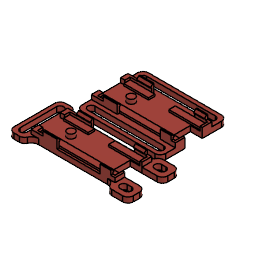
MicrophoneSenzor (Autodesk Fusion 360 design; units mm, degrees)
Autodesk Fusion 360 part; units mm, degrees
note: some values were not read from the file. Set by a fixed rule: which face or edge a step refers to.
sketch "Sketch1" plane through (0, 0, 0) normal (0, 0, 1) x (1, 0, 0)
  line L0 (0, 0) -> (36, 0)
  line L1 (36, 0) -> (36, 15)
  line L2 (36, 15) -> (0, 15)
  line L3 (0, 15) -> (0, 0)
  line L4 (36, 7.5) -> (20, 7.5) construction
  line L5 (36, 12) -> (32, 12)
  line L6 (32, 12) -> (32, 3)
  line L7 (32, 3) -> (36, 3)
  line L8 (36, 3) -> (36, 12)
  line L9 (36, 12) -> (32, 3) construction
  line L10 (32, 12) -> (36, 3) construction
  line L11 (0, 7.5) -> (8, 7.5) construction
  circle A0 centre (8, 7.5) radius 1.8
  point P0 (34, 7.5)
  dimension "d1" = 36
  dimension "d2" = 15
  dimension "d3" = 8
  dimension "d4" = 3.6
  constraint horizontal L0
  constraint vertical L1
  constraint horizontal L2
  constraint vertical L3
  constraint coincident L0.start L3.end
  constraint midpoint L1 L4.start
  constraint perpendicular L1 L4
  constraint horizontal L5
  constraint perpendicular L5 L6
  constraint parallel L5 L7
  constraint parallel L6 L8
  constraint coincident L9 P0
  constraint coincident L10 P0
  constraint coincident L1 L5.start
  constraint coincident L4 P0
  constraint midpoint L3 L11.start
  constraint perpendicular L3 L11
  constraint coincident L11.end A0.centre
  measures "d1" distance of L0.start L0.end
  measures "d2" distance of L0.start L2.end
  measures "d3" distance of L11.start L11.end
  measures "d4" diameter of A0
extrude "Extrude1" add sketch "Sketch1" along normal blind 1.6 contours L0 L1 L2 L3 L5 L6 L7 makes body 1
sketch "Sketch3" plane through (32, 0, 0) normal (1, 0, 0) x (0, 1, 0)
  line L0 (3, 0) -> (12, 0)
  line L1 (12, 0) -> (12, 1.6)
  line L2 (12, 1.6) -> (3, 1.6)
  line L3 (3, 1.6) -> (3, 0)
  circle A0 centre (7.5, 1.6) radius 3
  dimension "d7" = 6
  constraint midpoint L2 A0.centre
  measures "d7" diameter of A0
extrude "Extrude2" add sketch "Sketch3" along normal blind 5.5 contours L0 L2 A0 | L0 A0 | L2 A0 bodies 1
sketch "Sketch4" plane through (0, 0, 1.6) normal (0, 0, 1) x (-1, 0, 0)
  circle A0 centre (-8, -7.5) radius 1.8
  line L0 (-36, -12) -> (-36, -15)
  line L1 (-36, -15) -> (0, -15)
  line L2 (0, -15) -> (0, 0)
  line L3 (0, 0) -> (-36, 0)
  line L4 (-36, 0) -> (-36, -3)
  line L5 (-36, -3) -> (-32, -3)
  line L6 (-32, -3) -> (-32, -4.5)
  line L7 (-32, -4.5) -> (-32, -10.5)
  line L8 (-32, -10.5) -> (-32, -12)
  line L9 (-32, -12) -> (-36, -12)
  line L10 (0, -7.5) -> (-2.5, -7.5) construction
  line L11 (-2.5, -12.5) -> (0, -12.5)
  line L12 (0, -12.5) -> (0, -2.5)
  line L13 (0, -2.5) -> (-2.5, -2.5)
  line L14 (-2.5, -2.5) -> (-2.5, -12.5)
  line L15 (-2.5, -12.5) -> (0, -2.5) construction
  line L16 (0, -12.5) -> (-2.5, -2.5) construction
  circle A1 centre (-2.5, -10) radius 0.05
  circle A2 centre (0, -10) radius 0.05
  circle A3 centre (-2.5, -7.5) radius 0.05
  circle A4 centre (0, -7.5) radius 0.05
  circle A5 centre (-2.5, -5) radius 0.05
  circle A6 centre (0, -5) radius 0.05
  line L17 (-32, -9) -> (-29, -9)
  line L18 (-29, -9) -> (-29, -8.5)
  line L19 (-29, -8.5) -> (-32, -8.5)
  line L20 (-32, -8.5) -> (-32, -9)
  line L21 (-32, -6) -> (-29, -6)
  line L22 (-29, -6) -> (-29, -6.5)
  line L23 (-29, -6.5) -> (-32, -6.5)
  line L24 (-32, -6.5) -> (-32, -6)
  point P0 (-1.25, -7.5)
  dimension "d10" = 0.1
  dimension "d13" = 2.5
  dimension "d14" = 5
  constraint midpoint L2 L10.start
  constraint perpendicular L2 L10
  constraint horizontal L11
  constraint perpendicular L11 L12
  constraint parallel L11 L13
  constraint parallel L12 L14
  constraint coincident L15 P0
  constraint coincident L16 P0
  constraint midpoint L10 P0
  constraint coincident L14 A1.centre
  constraint horizontal L17
  constraint vertical L18
  constraint horizontal L19
  constraint vertical L20
  constraint coincident L7 L17.start
  constraint horizontal L21
  constraint vertical L22
  constraint horizontal L23
  constraint vertical L24
  constraint coincident L7 L21.start
  measures "d10" diameter of A1
extrude "Extrude3" add sketch "Sketch4" along normal blind 0.5 contours L7 L17 L18 L19 L20 | L7 L21 L22 L23 L24 bodies 1
extrude "Extrude4" add sketch "Sketch4" along normal blind 2.5 contours L2 L11 L12 L13 L14 A1 A2 A3 A4 A5 A6 bodies 1
sketch "Sketch5" plane through (0, 0, 1.6) normal (0, 0, 1) x (-1, 0, 0)
  line L0 (-2.5, -2.5) -> (0, -2.5)
  line L1 (0, -2.5) -> (0, 0)
  line L2 (0, 0) -> (-36, 0)
  line L3 (-36, 0) -> (-36, -3)
  line L4 (-36, -3) -> (-32, -3)
  line L5 (-32, -3) -> (-32, -4.5)
  line L6 (-32, -4.5) -> (-32, -6)
  line L7 (-32, -6) -> (-29, -6)
  line L8 (-29, -6) -> (-29, -6.5)
  line L9 (-29, -6.5) -> (-32, -6.5)
  line L10 (-32, -6.5) -> (-32, -8.5)
  line L11 (-32, -8.5) -> (-29, -8.5)
  line L12 (-29, -8.5) -> (-29, -9)
  line L13 (-29, -9) -> (-32, -9)
  line L14 (-32, -9) -> (-32, -10.5)
  line L15 (-32, -10.5) -> (-32, -12)
  line L16 (-32, -12) -> (-36, -12)
  line L17 (-36, -12) -> (-36, -15)
  line L18 (-36, -15) -> (0, -15)
  line L19 (0, -15) -> (0, -12.5)
  line L20 (0, -12.5) -> (-2.5, -12.5)
  line L21 (-2.5, -12.5) -> (-2.5, -10.05)
  arc A0 (-2.5, -10.05) -> (-2.5, -9.95) centre (-2.5, -10) ccw
  line L22 (-2.5, -9.95) -> (-2.5, -7.55)
  arc A1 (-2.5, -7.55) -> (-2.5, -7.45) centre (-2.5, -7.5) ccw
  line L23 (-2.5, -7.45) -> (-2.5, -5.05)
  arc A2 (-2.5, -5.05) -> (-2.5, -4.95) centre (-2.5, -5) ccw
  line L24 (-2.5, -4.95) -> (-2.5, -2.5)
  circle A3 centre (-8, -7.5) radius 1.8
  line L25 (-11.5, -15) -> (-21, -15)
  line L26 (-21, -15) -> (-21, -10.5)
  line L27 (-21, -10.5) -> (-11.5, -10.5)
  line L28 (-11.5, -10.5) -> (-11.5, -15)
  line L29 (-3.5, -14.5) -> (-6, -14.5)
  line L30 (-6, -14.5) -> (-6, -13.5)
  line L31 (-6, -13.5) -> (-3.5, -13.5)
  line L32 (-3.5, -13.5) -> (-3.5, -14.5)
  line L33 (-7.5, -13.5) -> (-7.5, -14.5)
  line L34 (-7.5, -14.5) -> (-10, -14.5)
  line L35 (-10, -14.5) -> (-10, -13.5)
  line L36 (-10, -13.5) -> (-7.5, -13.5)
  line L37 (-10, -1.5) -> (-10, -0.5)
  line L38 (-10, -0.5) -> (-7.5, -0.5)
  line L39 (-7.5, -0.5) -> (-7.5, -1.5)
  line L40 (-7.5, -1.5) -> (-10, -1.5)
  line L41 (-3.5, -0.5) -> (-3.5, -1.5)
  line L42 (-3.5, -1.5) -> (-6, -1.5)
  line L43 (-6, -0.5) -> (-3.5, -0.5)
  line L44 (-6, -1.5) -> (-6, -0.5)
  line L45 (-23, -13) -> (-25.5, -13)
  line L46 (-25.5, -13) -> (-25.5, -12)
  line L47 (-25.5, -12) -> (-23, -12)
  line L48 (-23, -12) -> (-23, -13)
  line L49 (-22, -10.5) -> (-24.5, -10.5)
  line L50 (-24.5, -10.5) -> (-24.5, -9.5)
  line L51 (-24.5, -9.5) -> (-22, -9.5)
  line L52 (-22, -9.5) -> (-22, -10.5)
  line L53 (-22, -3.5) -> (-24.5, -3.5)
  line L54 (-24.5, -3.5) -> (-24.5, -2.5)
  line L55 (-24.5, -2.5) -> (-22, -2.5)
  line L56 (-22, -2.5) -> (-22, -3.5)
  line L57 (-24.5, -1) -> (-22, -1)
  line L58 (-22, -1) -> (-22, -2)
  line L59 (-22, -2) -> (-24.5, -2)
  line L60 (-24.5, -2) -> (-24.5, -1)
  line L61 (-14, -6.5) -> (-18, -6.5)
  line L62 (-18, -6.5) -> (-18, -1.5)
  line L63 (-18, -1.5) -> (-14, -1.5)
  line L64 (-14, -1.5) -> (-14, -6.5)
  dimension "d19" = 9.5
  dimension "d20" = 4.5
  dimension "d21" = 2.5
  dimension "d22" = 1
  dimension "d23" = 2.5
  dimension "d24" = 1
  dimension "d25" = 2.5
  dimension "d26" = 1
  dimension "d27" = 2.5
  dimension "d28" = 1
  dimension "d29" = 2.5
  dimension "d30" = 1
  dimension "d31" = 2.5
  dimension "d32" = 1
  dimension "d33" = 2.5
  dimension "d34" = 1
  dimension "d35" = 2.5
  dimension "d36" = 1
  dimension "d37" = 4
  dimension "d38" = 5
  constraint horizontal L25
  constraint vertical L26
  constraint horizontal L27
  constraint vertical L28
  constraint horizontal L29
  constraint vertical L30
  constraint horizontal L31
  constraint vertical L32
  constraint horizontal L34
  constraint vertical L35
  constraint horizontal L36
  constraint vertical L33
  constraint horizontal L42
  constraint vertical L44
  constraint horizontal L43
  constraint vertical L41
  constraint horizontal L40
  constraint vertical L37
  constraint horizontal L38
  constraint vertical L39
  constraint horizontal L45
  constraint vertical L46
  constraint horizontal L47
  constraint vertical L48
  constraint horizontal L49
  constraint vertical L50
  constraint horizontal L51
  constraint vertical L52
  constraint horizontal L53
  constraint vertical L54
  constraint horizontal L55
  constraint vertical L56
  constraint horizontal L59
  constraint vertical L60
  constraint horizontal L57
  constraint vertical L58
  constraint horizontal L61
  constraint vertical L62
  constraint horizontal L63
  constraint vertical L64
  measures "d19" distance of L25.start L25.end
  measures "d20" distance of L25.start L27.end
  measures "d21" distance of L29.start L29.end
  measures "d22" distance of L29.start L31.end
  measures "d23" distance of L33.end L34.end
  measures "d24" distance of L33.end L33.start
  measures "d25" distance of L41.end L42.end
  measures "d26" distance of L41.end L41.start
  measures "d27" distance of L37.start L39.end
  measures "d28" distance of L39.end L38.end
  measures "d29" distance of L45.end L45.start
  measures "d30" distance of L45.start L47.end
  measures "d31" distance of L49.end L49.start
  measures "d32" distance of L49.start L51.end
  measures "d33" distance of L53.end L53.start
  measures "d34" distance of L53.start L55.end
  measures "d35" distance of L59.end L58.end
  measures "d36" distance of L58.end L57.end
  measures "d37" distance of L61.start L61.end
  measures "d38" distance of L61.start L63.end
extrude "Extrude5" add sketch "Sketch5" along normal blind 10.5 contours L18 L25 L26 L27 L28 bodies 1
extrude "Extrude6" add sketch "Sketch5" along normal blind 0.5 contours L29 L30 L31 L32 | L33 L34 L35 L36 | L37 L38 L39 L40 | L41 L42 L43 L44 | L45 L46 L47 L48 | L49 L50 L51 L52 | L53 L54 L55 L56 | L57 L58 L59 L60 bodies 1
extrude "Extrude7" add sketch "Sketch5" along normal blind 1 contours L61 L62 L63 L64 bodies 1
sketch "Sketch6" plane through (0, 0, 4.1) normal (0, 0, 1) x (-1, 0, 0)
  line L0 (0, -9.95) -> (0, -7.55)
  arc A0 (0, -7.45) -> (0, -7.55) centre (0, -7.5) ccw
  line L1 (0, -7.45) -> (0, -5.05)
  arc A1 (0, -4.95) -> (0, -5.05) centre (0, -5) ccw
  line L2 (0, -4.95) -> (0, -2.5)
  line L3 (0, -2.5) -> (-2.5, -2.5)
  line L4 (-2.5, -2.5) -> (-2.5, -4.95)
  arc A2 (-2.5, -5.05) -> (-2.5, -4.95) centre (-2.5, -5) ccw
  line L5 (-2.5, -5.05) -> (-2.5, -7.45)
  arc A3 (-2.5, -7.55) -> (-2.5, -7.45) centre (-2.5, -7.5) ccw
  line L6 (-2.5, -7.55) -> (-2.5, -9.95)
  arc A4 (-2.5, -10.05) -> (-2.5, -9.95) centre (-2.5, -10) ccw
  line L7 (-2.5, -10.05) -> (-2.5, -12.5)
  line L8 (-2.5, -12.5) -> (0, -12.5)
  line L9 (0, -12.5) -> (0, -10.05)
  arc A5 (0, -9.95) -> (0, -10.05) centre (0, -10) ccw
  line L10 (-1, -11.5) -> (-1.5, -11.5)
  line L11 (-1.5, -11.5) -> (-1.5, -11)
  line L12 (-1.5, -11) -> (-1, -11)
  line L13 (-1, -11) -> (-1, -11.5)
  line L14 (-1, -9) -> (-1.5, -9)
  line L15 (-1.5, -9) -> (-1.5, -8.5)
  line L16 (-1.5, -8.5) -> (-1, -8.5)
  line L17 (-1, -8.5) -> (-1, -9)
  line L18 (-1, -6.5) -> (-1.5, -6.5)
  line L19 (-1.5, -6.5) -> (-1.5, -6)
  line L20 (-1.5, -6) -> (-1, -6)
  line L21 (-1, -6) -> (-1, -6.5)
  line L22 (-1, -4) -> (-1.5, -4)
  line L23 (-1.5, -4) -> (-1.5, -3.5)
  line L24 (-1.5, -3.5) -> (-1, -3.5)
  line L25 (-1, -3.5) -> (-1, -4)
  dimension "d47" = 0
  dimension "d48" = 7.5
  constraint horizontal L10
  constraint vertical L11
  constraint horizontal L12
  constraint vertical L13
extrude "Extrude8" add sketch "Sketch6" along normal blind 1.5 contours L10 L11 L12 L13 | L14 L15 L16 L17 | L18 L19 L20 L21 | L22 L23 L24 L25 bodies 1
sketch "Sketch7" plane through (1, 0, 0) normal (-1, 0, 0) x (0, -1, 0)
  line L0 (-11.5, 4.1) -> (-11, 4.1)
  line L1 (-11, 4.1) -> (-11, 5.6)
  line L2 (-11, 5.6) -> (-11.5, 5.6)
  line L3 (-11.5, 5.6) -> (-11.5, 4.1)
  line L4 (-11, 5.6) -> (-11.5, 5.6)
  line L5 (-11.5, 5.6) -> (-11.5, 5.1)
  line L6 (-11.5, 5.1) -> (-11, 5.1)
  line L7 (-11, 5.1) -> (-11, 5.6)
  line L8 (-9, 5.6) -> (-9, 5.1)
  line L9 (-9, 5.1) -> (-8.5, 5.1)
  line L10 (-8.5, 5.6) -> (-9, 5.6)
  line L11 (-8.5, 5.1) -> (-8.5, 5.6)
  line L12 (-6.5, 5.6) -> (-6.5, 5.1)
  line L13 (-6.5, 5.1) -> (-6, 5.1)
  line L14 (-6, 5.6) -> (-6.5, 5.6)
  line L15 (-6, 5.1) -> (-6, 5.6)
  line L16 (-4, 5.6) -> (-4, 5.1)
  line L17 (-4, 5.1) -> (-3.5, 5.1)
  line L18 (-3.5, 5.6) -> (-4, 5.6)
  line L19 (-3.5, 5.1) -> (-3.5, 5.6)
  dimension "d51" = 0.5
  dimension "d54" = 7.5
  dimension "d55" = 0
  constraint horizontal L4
  constraint vertical L5
  constraint horizontal L6
  constraint vertical L7
  constraint coincident L1.end L2.start
  measures "d51" distance of L1.end L6.end
extrude "Extrude9" add sketch "Sketch7" along normal blind 7 contours L1 L2 L3 L4 L5 L6 L7 | L8 L9 L10 L11 | L12 L13 L14 L15 | L16 L17 L18 L19 bodies 1
sketch "Sketch8" plane through (0, 0, 12.1) normal (0, 0, 1) x (-1, 0, 0)
  line L0 (-11.5, -10.5) -> (-21, -10.5)
  line L1 (-21, -10.5) -> (-21, -15)
  line L2 (-21, -15) -> (-11.5, -15)
  line L3 (-11.5, -15) -> (-11.5, -10.5)
  circle A0 centre (-12.5, -14) radius 1
  constraint tangent L2 A0
extrude "Extrude10" add sketch "Sketch8" along normal blind 1 contours A0 bodies 1
sketch "Sketch10" plane through (0, 0, 0) normal (0, 0, 1) x (1, 0, 0)
  line L0 (-2, 17) -> (37, 17)
  line L1 (37, 17) -> (37, -2)
  line L2 (37, -2) -> (-2, -2)
  line L3 (-2, -2) -> (-2, 17)
  line L4 (37, 11.5) -> (31.5, 11.5)
  line L5 (31.5, 11.5) -> (31.5, 3.5)
  line L6 (31.5, 3.5) -> (37, 3.5)
  line L7 (37, 3.5) -> (37, 11.5)
  constraint horizontal L0
  constraint vertical L1
  constraint horizontal L2
  constraint vertical L3
  constraint horizontal L4
  constraint vertical L5
  constraint horizontal L6
  constraint vertical L7
  constraint coincident L1 L4.start
sketch "Sketch11" plane through (0, 0, 0) normal (0, 0, -1) x (1, 0, 0)
  circle A0 centre (8, -7.5) radius 1.8
  line L0 (36, -15) -> (36, -12)
  line L1 (36, -12) -> (32, -12)
  line L2 (32, -12) -> (32, -10.0377)
  line L3 (32, -10.0377) -> (32, -4.9623)
  line L4 (32, -4.9623) -> (32, -3)
  line L5 (32, -3) -> (36, -3)
  line L6 (36, -3) -> (36, 0)
  line L7 (36, 0) -> (0, 0)
  line L8 (0, 0) -> (0, -15)
  line L9 (0, -15) -> (36, -15)
  circle A1 centre (1.25, -3.75) radius 0.3536
  circle A2 centre (1.25, -6.25) radius 0.3536
  circle A3 centre (1.25, -8.75) radius 0.3536
  circle A4 centre (1.25, -11.25) radius 0.3536
  circle A5 centre (14.75, -13.75) radius 0.3536
  circle A6 centre (16.25, -13.75) radius 0.3536
  circle A7 centre (17.75, -13.75) radius 0.3536
  circle A8 centre (29.25, -6.25) radius 0.3536
  circle A9 centre (29.25, -8.75) radius 0.3536
extrude "Extrude11" add sketch "Sketch11" along normal blind 0.5 draft -30 contours A1 | A2 | A3 | A4 | A5 | A6 | A7 | A8 | A9 bodies 1
move_body "Move1" bodies 1 to x (1, 0, 0) y (0, 1, 0) z (0, 0, 1) at (0, 0, 1)
extrude "Extrude12" add sketch "Sketch10" against normal blind 2.5 separate body contours L0 L1 L2 L3 L4 L5 L6 makes body 2
sketch "Sketch12" plane through (0, 0, 0) normal (0, 0, 1) x (-1, 0, 0)
  line L0 (-31.5, -3.5) -> (-31.5, -11.5)
  line L1 (-31.5, -11.5) -> (-37, -11.5)
  line L2 (-37, -11.5) -> (-37, -17)
  line L3 (-37, -17) -> (2, -17)
  line L4 (2, -17) -> (2, 2)
  line L5 (2, 2) -> (-37, 2)
  line L6 (-37, 2) -> (-37, -3.5)
  line L7 (-37, -3.5) -> (-31.5, -3.5)
  line L8 (-36, -15) -> (-21, -15)
  line L9 (-21, -15) -> (-21, -12)
  line L10 (-21, -12) -> (-36, -12)
  line L11 (-36, -12) -> (-36, -15)
  line L12 (-36, 0) -> (-21, 0)
  line L13 (-21, -3) -> (-36, -3)
  line L14 (-36, -3) -> (-36, 0)
  line L15 (0, 0) -> (-21, 0)
  line L16 (-21, -3) -> (0, -3)
  line L17 (0, -3) -> (0, 0)
  line L18 (0, -15) -> (-11.5, -15)
  line L19 (-11.5, -15) -> (-11.5, -12)
  line L20 (-11.5, -12) -> (0, -12)
  line L21 (0, -12) -> (0, -15)
  circle A0 centre (-8, -7.5) radius 1.75
  dimension "d64" = 3.5
  constraint horizontal L8
  constraint vertical L9
  constraint horizontal L10
  constraint vertical L11
  constraint horizontal L12
  constraint horizontal L13
  constraint vertical L14
  constraint horizontal L15
  constraint horizontal L16
  constraint vertical L17
  constraint coincident L15.start L17.end
  constraint horizontal L18
  constraint vertical L19
  constraint horizontal L20
  constraint vertical L21
  measures "d64" diameter of A0
extrude "Extrude13" add sketch "Sketch12" along normal blind 1 contours L8 L9 L10 L11 | L12 L13 L14 L15 L16 L17 | L18 L19 L20 L21 bodies 2
sketch "Sketch13" plane through (0, 0, 0) normal (0, 0, 1) x (-1, 0, 0)
  line L0 (-36, -12) -> (-21, -12)
  line L1 (-21, -12) -> (-21, -15)
  line L2 (-21, -15) -> (-36, -15)
  line L3 (-36, -15) -> (-36, -12)
  line L4 (0, -12) -> (0, -15)
  line L5 (0, -15) -> (-11.5, -15)
  line L6 (-11.5, -15) -> (-11.5, -12)
  line L7 (-11.5, -12) -> (0, -12)
  line L8 (-36, -3) -> (-36, 0)
  line L9 (-36, 0) -> (0, 0)
  line L10 (0, 0) -> (0, -3)
  line L11 (0, -3) -> (-36, -3)
  line L12 (-31.5, -3.5) -> (-31.5, -11.5)
  line L13 (-31.5, -11.5) -> (-37, -11.5)
  line L14 (-37, -11.5) -> (-37, -17)
  line L15 (-37, -17) -> (2, -17)
  line L16 (2, -17) -> (2, 2)
  line L17 (2, 2) -> (-37, 2)
  line L18 (-37, 2) -> (-37, -3.5)
  line L19 (-37, -3.5) -> (-31.5, -3.5)
  line L20 (-35, 2) -> (-30, 2)
  line L21 (-30, 2) -> (-30, 0)
  line L22 (-30, 0) -> (-35, 0)
  line L23 (-35, 0) -> (-35, 2)
  line L24 (-10, 2) -> (-3.5, 2)
  line L25 (-3.5, 2) -> (-3.5, 0)
  line L26 (-3.5, 0) -> (-10, 0)
  line L27 (-10, 0) -> (-10, 2)
  line L28 (2, -7.5) -> (-32, -7.5) construction
  line L29 (-3.5, -17) -> (-3.5, -15)
  line L30 (-3.5, -15) -> (-10, -15)
  line L31 (-10, -17) -> (-3.5, -17)
  line L32 (-10, -15) -> (-10, -17)
  line L33 (-35, -15) -> (-35, -17)
  line L34 (-35, -17) -> (-30, -17)
  line L35 (-30, -15) -> (-35, -15)
  line L36 (-30, -17) -> (-30, -15)
  constraint horizontal L20
  constraint vertical L21
  constraint horizontal L22
  constraint vertical L23
  constraint coincident L9 L21.end
  constraint coincident L17 L20.start
  constraint horizontal L24
  constraint vertical L25
  constraint horizontal L26
  constraint vertical L27
  constraint coincident L9 L25.end
  constraint coincident L17 L24.start
  constraint midpoint L16 L28.start
  constraint perpendicular L12 L28
  constraint symmetric L20.start L28 L33.end
  constraint symmetric L20.end L28 L34.end
  constraint symmetric L21.end L28 L35.start
  constraint symmetric L22.end L28 L33.start
  constraint symmetric L24.start L28 L31.start
  constraint symmetric L24.end L28 L29.start
  constraint symmetric L25.end L28 L29.end
  constraint symmetric L26.end L28 L30.end
extrude "Extrude14" add sketch "Sketch13" sketch "Sketch12" along normal blind 4 contours L2 L15 L33 L34 L35 L36 | L5 L15 L29 L30 L31 L32 | L9 L17 L24 L25 L26 L27 | L9 L17 L20 L21 L22 L23 of sketch 2 contours A0 bodies 2
sketch "Sketch14" plane through (0, 0, 4) normal (0, 0, 1) x (-1, 0, 0)
  line L0 (-10, 0) -> (-3.5, 0)
  line L1 (-3.5, 0) -> (-3.5, 2)
  line L2 (-3.5, 2) -> (-10, 2)
  line L3 (-10, 2) -> (-10, 0)
  line L4 (-3.5, -0.5) -> (-10, -0.5)
  line L5 (-10, -0.5) -> (-10, 0)
  line L6 (-10, 0) -> (-3.5, 0)
  line L7 (-3.5, 0) -> (-3.5, -0.5)
  line L8 (-35, 0) -> (-30, 0)
  line L9 (-30, 0) -> (-30, -0.5)
  line L10 (-30, -0.5) -> (-35, -0.5)
  line L11 (-35, -0.5) -> (-35, 0)
  line L12 (-32, 0) -> (-32, -15) construction
  line L13 (-32, -15) -> (-32, -7.5) construction
  line L14 (-5, -7.5) -> (-32, -7.5) construction
  line L15 (-10, -15) -> (-3.5, -15)
  line L16 (-3.5, -15) -> (-3.5, -14.5)
  line L17 (-3.5, -14.5) -> (-10, -14.5)
  line L18 (-10, -14.5) -> (-10, -15)
  line L19 (-35, -15) -> (-30, -15)
  line L20 (-30, -15) -> (-30, -14.5)
  line L21 (-35, -14.5) -> (-35, -15)
  line L22 (-30, -14.5) -> (-35, -14.5)
  constraint horizontal L4
  constraint vertical L5
  constraint horizontal L6
  constraint vertical L7
  constraint coincident L0.start L3.end
  constraint horizontal L8
  constraint vertical L9
  constraint horizontal L10
  constraint vertical L11
  constraint coincident L8 L12.start
  constraint perpendicular L10 L12
  constraint midpoint L12 L13.end
  constraint perpendicular L13 L14
  constraint symmetric L4.start L14 L16.end
  constraint symmetric L4.end L14 L17.end
  constraint symmetric L0.start L14 L15.start
  constraint symmetric L0.end L14 L15.end
  constraint symmetric L8.start L14 L19.start
  constraint symmetric L8.end L14 L19.end
  constraint symmetric L9.end L14 L20.end
  constraint symmetric L10.end L14 L21.start
extrude "Extrude15" add sketch "Sketch14" against normal blind 1.3 contours L0 L4 L5 L6 L7 | L8 L9 L10 L11 | L15 L16 L17 L18 | L19 L20 L21 L22 bodies 2
chamfer "Chamfer1" distance 1 angle 45 4 edges at (6.75, 14.5, 4) (6.75, 0.5, 4) (32.5, 0.5, 4) (32.5, 14.5, 4) on bodies 2
sketch "Sketch15" plane through (0, 0, 0) normal (0, 0, 1) x (-1, 0, 0)
  line L0 (0, -2.5) -> (2, -2.5)
  line L1 (2, -2.5) -> (2, 2)
  line L2 (2, 2) -> (0, 2)
  line L3 (0, 0) -> (0, -2.5)
  line L4 (-3.5, 2) -> (0, 2)
  line L5 (0, 0) -> (-3.5, 0)
  line L6 (-3.5, 0) -> (-3.5, 2)
  line L7 (0, -12.5) -> (2, -12.5)
  line L8 (2, -12.5) -> (2, -17)
  line L9 (2, -17) -> (0, -17)
  line L10 (0, -15) -> (0, -12.5)
  line L11 (-3.5, -17) -> (0, -17)
  line L12 (0, -15) -> (-3.5, -15)
  line L13 (-3.5, -15) -> (-3.5, -17)
  line L14 (-35, 2) -> (-37, 2)
  line L15 (-37, 2) -> (-37, 0)
  line L16 (-36, 0) -> (-35, 0)
  line L17 (-35, 0) -> (-35, 2)
  line L18 (-37, -3.5) -> (-36, -3.5)
  line L19 (-36, -3.5) -> (-36, 0)
  line L20 (-37, 0) -> (-37, -3.5)
  line L21 (-37, -11.5) -> (-36, -11.5)
  line L22 (-36, -11.5) -> (-36, -15)
  line L23 (-37, -15) -> (-37, -11.5)
  line L24 (-35, -17) -> (-37, -17)
  line L25 (-37, -17) -> (-37, -15)
  line L26 (-36, -15) -> (-35, -15)
  line L27 (-35, -15) -> (-35, -17)
  constraint horizontal L0
  constraint vertical L1
  constraint horizontal L2
  constraint vertical L3
  constraint horizontal L4
  constraint horizontal L5
  constraint vertical L6
  constraint coincident L3.start L5.start
  constraint coincident L5 L3.start
  constraint horizontal L7
  constraint vertical L8
  constraint horizontal L9
  constraint vertical L10
  constraint horizontal L11
  constraint horizontal L12
  constraint vertical L13
  constraint horizontal L14
  constraint vertical L15
  constraint horizontal L16
  constraint vertical L17
  constraint horizontal L18
  constraint vertical L19
  constraint vertical L20
  constraint horizontal L21
  constraint vertical L22
  constraint vertical L23
  constraint horizontal L24
  constraint vertical L25
  constraint horizontal L26
  constraint vertical L27
extrude "Extrude16" add sketch "Sketch15" along normal blind 2 bodies 2
copy_body "CopyPasteBodies1" bodies 2 makes body 3
sketch "Sketch16" plane through (0, 0, -2.5) normal (0, 0, -1) x (1, 0, 0)
  line L0 (31.5, -11.5) -> (31.5, -3.5)
  line L1 (31.5, -3.5) -> (37, -3.5)
  line L2 (37, -3.5) -> (37, 2)
  line L3 (37, 2) -> (-2, 2)
  line L4 (-2, 2) -> (-2, -17)
  line L5 (-2, -17) -> (37, -17)
  line L6 (37, -17) -> (37, -11.5)
  line L7 (37, -11.5) -> (31.5, -11.5)
  line L8 (-2, 2) -> (37, 2) construction
  line L9 (37, -3.5) -> (37, -17) construction
  line L10 (37, -17) -> (-2, -17) construction
  line L11 (-2, -17) -> (-2, 2) construction
  line L12 (17.5, -7.5) -> (-5.5, -7.5) construction
  line L13 (-5.5, -7.5) -> (42.5, -7.5) construction
  line L14 (42.5, -7.5) -> (42.5, -15.5) construction
  line L15 (42.5, -15.5) -> (42.5, 0.5) construction
  line L16 (-9, -7.5) -> (-9, -17)
  line L17 (-2, -17) -> (-2, -7.5)
  line L18 (-9, -7.5) -> (-9, 2)
  line L19 (-6.5, 4.5) -> (-2, 4.5)
  line L20 (-2, 2) -> (-2, -7.5)
  line L21 (-7.15, 1) -> (-7.15, -16)
  arc A0 (-7.15, -16) -> (-3.85, -16) centre (-5.5, -16) ccw
  line L22 (-3.85, -16) -> (-3.85, 1)
  arc A1 (-3.85, 1) -> (-7.15, 1) centre (-5.5, 1) ccw
  line L23 (-5.5, 1) -> (-5.5, -16) construction
  line L24 (44, -3.5) -> (38.5, -3.5)
  line L25 (38.5, 4.5) -> (44, 4.5)
  line L26 (46.5, 2) -> (46.5, -1)
  line L27 (46.5, -3.5) -> (38.5, 4.5) construction
  line L28 (38.5, -3.5) -> (46.5, 4.5) construction
  line L29 (46.5, -14) -> (46.5, -17)
  line L30 (46.5, -19.5) -> (38.5, -11.5) construction
  line L31 (38.5, -19.5) -> (46.5, -11.5) construction
  line L32 (38.5, 4.5) -> (-2, 4.5)
  line L33 (37, -3.5) -> (38.5, -3.5)
  arc A2 (-9, -17) -> (-6.5, -19.5) centre (-6.5, -17) ccw
  arc A3 (-6.5, 4.5) -> (-9, 2) centre (-6.5, 2) ccw
  arc A4 (46.5, 2) -> (44, 4.5) centre (44, 2) ccw
  arc A5 (44, -3.5) -> (46.5, -1) centre (44, -1) ccw
  arc A6 (46.5, -14) -> (44, -11.5) centre (44, -14) ccw
  arc A7 (44, -19.5) -> (46.5, -17) centre (44, -17) ccw
  line L34 (44, -11.5) -> (37, -11.5)
  line L35 (44, -19.5) -> (-6.5, -19.5)
  line L36 (42.5, 2.15) -> (40.5, 2.15)
  arc A8 (40.5, 2.15) -> (40.5, -1.15) centre (40.5, 0.5) ccw
  line L37 (40.5, -1.15) -> (42.5, -1.15)
  arc A9 (42.5, -1.15) -> (42.5, 2.15) centre (42.5, 0.5) ccw
  line L38 (42.5, 0.5) -> (40.5, 0.5) construction
  line L39 (42.5, -13.85) -> (40.5, -13.85)
  arc A10 (40.5, -13.85) -> (40.5, -17.15) centre (40.5, -15.5) ccw
  line L40 (40.5, -17.15) -> (42.5, -17.15)
  arc A11 (42.5, -17.15) -> (42.5, -13.85) centre (42.5, -15.5) ccw
  arc A12 (42.5, -17.15) -> (42.5, -13.85) centre (42.5, -15.5) ccw
  arc A13 (42.5, -1.15) -> (42.5, 2.15) centre (42.5, 0.5) ccw
  point P0 (-5.5, -7.5)
  point P1 (42.5, 0.5)
  point P2 (42.5, -15.5)
  dimension "d74" = 3.3
  dimension "d75" = 17
  dimension "d76" = 7
  dimension "d77" = 7
  dimension "d78" = 3.3
  dimension "d79" = 3.3
  dimension "d80" = 8
  dimension "d81" = 8
  dimension "d84" = 2.5
  constraint horizontal L8
  constraint vertical L9
  constraint horizontal L10
  constraint vertical L11
  constraint coincident L5.end L6.start
  constraint coincident L3.end L4.start
  constraint perpendicular L4 L12
  constraint perpendicular L9 L13
  constraint perpendicular L13 L14
  constraint perpendicular L13 L15
  constraint vertical L16
  constraint vertical L17
  constraint midpoint L4 L17.end
  constraint vertical L18
  constraint horizontal L19
  constraint vertical L20
  constraint tangent L21 A0
  constraint tangent A0 L22
  constraint parallel L21 L22
  constraint tangent L22 A1
  constraint tangent L21 A1
  constraint perpendicular L12 L23
  constraint coincident P0 L12.end
  constraint midpoint L23 P0
  constraint coincident P2 L14.end
  constraint coincident P1 L15.end
  constraint horizontal L24
  constraint parallel L24 L25
  constraint coincident L27 P1
  constraint coincident L28 P1
  constraint coincident L30 P2
  constraint coincident L31 P2
  constraint perpendicular L20 L32
  constraint coincident L1.end L2.start
  constraint tangent L16 A2
  constraint tangent L18 A3
  constraint tangent L19 A3
  constraint equal A2 A3
  constraint coincident L28.end L26
  constraint coincident L28.end L25
  constraint tangent L26 A4
  constraint tangent L25 A4
  constraint equal A2 A4
  constraint coincident L27.start L24
  constraint coincident L27.start L26
  constraint tangent L24 A5
  constraint tangent L26 A5
  constraint equal A2 A5
  constraint coincident L31.end L29
  constraint tangent L29 A6
  constraint equal A2 A6
  constraint coincident L30.start L29
  constraint tangent L29 A7
  constraint equal A2 A7
  constraint coincident L6.end L7.start
  constraint tangent A2 L35
  constraint tangent L36 A8
  constraint tangent A8 L37
  constraint parallel L36 L37
  constraint tangent L37 A9
  constraint tangent L36 A9
  constraint horizontal L38
  constraint tangent L39 A10
  constraint tangent A10 L40
  constraint parallel L39 L40
  constraint tangent L40 A11
  constraint tangent L39 A11
  measures "d74" diameter of A0
  measures "d75" distance of A1.centre A0.centre
  measures "d76" distance of L16 L17
  measures "d77" distance of L18 L20
  measures "d78" diameter of A12
  measures "d79" diameter of A13
  measures "d80" distance of L30.end L31.end
  measures "d81" distance of L31.start L30.end
  measures "d84" radius of A2
extrude "Extrude17" add sketch "Sketch16" against normal blind 2.5 contours L2 L3 L4 L5 L6 L16 L17 L18 L19 L20 L24 L25 L26 L29 L32 L33 A2 A3 A4 A5 A6 A7 L34 L35 bodies 2
sketch "Sketch17" plane through (0, 0, -2.5) normal (0, 0, -1) x (1, 0, 0)
  line L0 (31.5, -11.5) -> (31.5, -3.5)
  line L1 (31.5, -3.5) -> (37, -3.5)
  line L2 (37, -3.5) -> (37, 2)
  line L3 (37, 2) -> (-2, 2)
  line L4 (-2, 2) -> (-2, -17)
  line L5 (-2, -17) -> (37, -17)
  line L6 (37, -17) -> (37, -11.5)
  line L7 (37, -11.5) -> (31.5, -11.5)
  line L8 (-2, -17) -> (37, -17) construction
  line L9 (37, -17) -> (37, 2) construction
  line L10 (37, 2) -> (-2, 2) construction
  line L11 (-2, 2) -> (-2, -17) construction
  line L12 (37, -7.5) -> (-2, -7.5) construction
  line L13 (17.5, -7.5) -> (17.5, -17) construction
  line L14 (17.5, 2) -> (17.5, -7.5) construction
  line L15 (17.5, -7.5) -> (17.5, -19.5) construction
  line L16 (17.5, -19.5) -> (17.5, 4.5) construction
  line L17 (-2, 2) -> (37, 2)
  line L18 (37, 2) -> (37, 5.5)
  line L19 (34.5, 8) -> (0.5, 8)
  line L20 (-2, 5.5) -> (-2, 2)
  line L21 (-2, -17) -> (37, -17)
  line L22 (37, -17) -> (37, -20.5)
  line L23 (34.5, -23) -> (0.5, -23)
  line L24 (-2, -20.5) -> (-2, -17)
  line L25 (1.5, -21.15) -> (33.5, -21.15)
  arc A0 (33.5, -21.15) -> (33.5, -17.85) centre (33.5, -19.5) ccw
  line L26 (33.5, -17.85) -> (1.5, -17.85)
  arc A1 (1.5, -17.85) -> (1.5, -21.15) centre (1.5, -19.5) ccw
  line L27 (1.5, -19.5) -> (33.5, -19.5) construction
  line L28 (1.5, 6.15) -> (33.5, 6.15)
  arc A2 (33.5, 2.85) -> (33.5, 6.15) centre (33.5, 4.5) ccw
  arc A3 (1.5, 6.15) -> (1.5, 2.85) centre (1.5, 4.5) ccw
  line L29 (33.5, 2.85) -> (1.5, 2.85)
  line L30 (-2, 5.5) -> (-2, 2)
  line L31 (-2, 2) -> (37, 2)
  line L32 (34.5, 8) -> (0.5, 8)
  line L33 (37, 2) -> (37, 5.5)
  arc A4 (34.5, -23) -> (37, -20.5) centre (34.5, -20.5) ccw
  arc A5 (-2, -20.5) -> (0.5, -23) centre (0.5, -20.5) ccw
  arc A6 (0.5, 8) -> (-2, 5.5) centre (0.5, 5.5) ccw
  arc A7 (37, 5.5) -> (34.5, 8) centre (34.5, 5.5) ccw
  point P0 (17.5, -19.5)
  dimension "d85" = 3.3
  dimension "d86" = 2.5
  constraint horizontal L8
  constraint vertical L9
  constraint horizontal L10
  constraint vertical L11
  constraint coincident L2.end L3.start
  constraint coincident L4.end L5.start
  constraint midpoint L9 L12.start
  constraint perpendicular L9 L12
  constraint midpoint L12 L13.start
  constraint perpendicular L12 L13
  constraint midpoint L3 L14.start
  constraint perpendicular L12 L14
  constraint perpendicular L12 L15
  constraint perpendicular L3 L16
  constraint horizontal L17
  constraint vertical L18
  constraint horizontal L19
  constraint vertical L20
  constraint horizontal L21
  constraint vertical L22
  constraint horizontal L23
  constraint vertical L24
  constraint tangent L25 A0
  constraint tangent A0 L26
  constraint parallel L25 L26
  constraint tangent L26 A1
  constraint tangent L25 A1
  constraint perpendicular L15 L27
  constraint coincident P0 L15.end
  constraint midpoint L27 P0
  constraint symmetric L4.end L12 L3.end
  constraint symmetric L12 L5.end L2.end
  constraint symmetric L12 L25.start L28.start
  constraint symmetric L12 L25.end L28.end
  constraint symmetric L12 A0.end A2.start
  constraint symmetric L12 L26.end A3.end
  constraint symmetric L12 A0 A2
  constraint symmetric L12 A1 A3
  constraint tangent L22 A4
  constraint tangent L23 A4
  constraint tangent L23 A5
  constraint tangent L24 A5
  constraint equal A4 A5
  constraint tangent L30 A6
  constraint tangent L32 A6
  constraint equal A4 A6
  constraint tangent L32 A7
  constraint tangent L33 A7
  constraint equal A4 A7
  measures "d85" diameter of A0
  measures "d86" radius of A4
extrude "Extrude18" add sketch "Sketch17" against normal blind 2.5 contours L5 L21 L22 L23 L24 A4 A5 | L3 L17 L18 L19 L20 L30 L31 L32 L33 A6 A7 bodies 3
extrude "Extrude19" cut 2 faces at (7.8333, -2, 2) (31.6667, -2, 2) along direction (0, 1, 0) blind 1 on bodies 3 bodies 3
extrude "Extrude20" cut 2 faces at (7.8333, 17, 2) (31.6667, 17, 2) along direction (0, -1, 0) blind 1 on bodies 3 bodies 3
extrude "Extrude21" cut 3 faces at (15.3333, 2, 1) (7.1667, 13, 1) (29, 13, 1) along direction (0, 0, -1) blind 0.1 on bodies 2 bodies 2 3
extrude "Extrude22" cut 2 faces at (31.6667, 17, 2) (7.8333, 17, 2) along direction (0, -1, 0) blind 1 on bodies 2 bodies 2
extrude "Extrude23" cut 2 faces at (31.6667, -2, 2) (7.8333, -2, 2) along direction (0, 1, 0) blind 1 on bodies 2 bodies 2
extrude "Extrude24" cut 1 faces at (8.5895, 7.1876, 4) along direction (0, 0, -1) blind 2 on bodies 3 bodies 2 3
sketch "Sketch18" plane through (0, 0, 0) normal (0, 0, 1) x (-1, 0, 0)
  line L0 (-10, -16) -> (-10, -15)
  line L1 (-10, -15) -> (-11.5, -15)
  line L2 (-11.5, -15) -> (-11.5, -12)
  line L3 (-11.5, -12) -> (0, -12)
  line L4 (0, -12) -> (0, -12.5)
  line L5 (0, -12.5) -> (2, -12.5)
  line L6 (2, -12.5) -> (2, -16)
  line L7 (2, -16) -> (-10, -16)
  arc A0 (-42.5, 2.15) -> (-42.5, -1.15) centre (-42.5, 0.5) ccw
  line L8 (-42.5, 2.15) -> (-40.5, 2.15)
  arc A1 (-40.5, -1.15) -> (-40.5, 2.15) centre (-40.5, 0.5) ccw
  line L9 (-40.5, -1.15) -> (-42.5, -1.15)
  arc A2 (-42.5, -13.85) -> (-42.5, -17.15) centre (-42.5, -15.5) ccw
  line L10 (-42.5, -13.85) -> (-40.5, -13.85)
  arc A3 (-40.5, -17.15) -> (-40.5, -13.85) centre (-40.5, -15.5) ccw
  line L11 (-40.5, -17.15) -> (-42.5, -17.15)
  arc A4 (7.15, 1) -> (3.85, 1) centre (5.5, 1) ccw
  line L12 (7.15, 1) -> (7.15, -16)
  arc A5 (3.85, -16) -> (7.15, -16) centre (5.5, -16) ccw
  line L13 (3.85, -16) -> (3.85, 1)
  line L14 (-30, -16) -> (-37, -16)
  line L15 (-37, -16) -> (-37, -11.5)
  line L16 (-37, -11.5) -> (-44, -11.5)
  arc A6 (-44, -11.5) -> (-46.5, -14) centre (-44, -14) ccw
  line L17 (-46.5, -14) -> (-46.5, -17)
  arc A7 (-46.5, -17) -> (-44, -19.5) centre (-44, -17) ccw
  line L18 (-44, -19.5) -> (6.5, -19.5)
  arc A8 (6.5, -19.5) -> (9, -17) centre (6.5, -17) ccw
  line L19 (9, -17) -> (9, 2)
  arc A9 (9, 2) -> (6.5, 4.5) centre (6.5, 2) ccw
  line L20 (6.5, 4.5) -> (-44, 4.5)
  arc A10 (-44, 4.5) -> (-46.5, 2) centre (-44, 2) ccw
  line L21 (-46.5, 2) -> (-46.5, -1)
  arc A11 (-46.5, -1) -> (-44, -3.5) centre (-44, -1) ccw
  line L22 (-44, -3.5) -> (-37, -3.5)
  line L23 (-37, -3.5) -> (-37, 1)
  line L24 (-37, 1) -> (-30, 1)
  line L25 (-30, 1) -> (-30, 0)
  line L26 (-30, 0) -> (-10, 0)
  line L27 (-10, 0) -> (-10, 1)
  line L28 (-10, 1) -> (2, 1)
  line L29 (2, 1) -> (2, -2.5)
  line L30 (2, -2.5) -> (0, -2.5)
  line L31 (0, -2.5) -> (0, -3)
  line L32 (0, -3) -> (-36, -3)
  line L33 (-36, -3) -> (-36, -3.5)
  line L34 (-36, -3.5) -> (-31.5, -3.5)
  line L35 (-31.5, -3.5) -> (-31.5, -11.5)
  line L36 (-31.5, -11.5) -> (-36, -11.5)
  line L37 (-36, -11.5) -> (-36, -12)
  line L38 (-36, -12) -> (-21, -12)
  line L39 (-21, -12) -> (-21, -15)
  line L40 (-21, -15) -> (-30, -15)
  line L41 (-30, -15) -> (-30, -16)
  circle A12 centre (-8, -7.5) radius 1.75
  line L42 (2, -16) -> (-37, -16)
  line L43 (-37, -16) -> (-37, -19.5)
  line L44 (-37, -19.5) -> (2, -19.5)
  line L45 (2, -19.5) -> (2, -16)
  line L46 (2, 1) -> (-37, 1)
  line L47 (-37, 1) -> (-37, 4.5)
  line L48 (-37, 4.5) -> (2, 4.5)
  line L49 (2, 4.5) -> (2, 1)
  constraint horizontal L42
  constraint vertical L43
  constraint horizontal L44
  constraint vertical L45
  constraint coincident L18 L43.end
  constraint coincident L6.end L7.start
  constraint horizontal L46
  constraint vertical L47
  constraint horizontal L48
  constraint vertical L49
  constraint coincident L20 L47.end
  constraint coincident L28.end L29.start
extrude "Extrude25" cut sketch "Sketch18" against normal blind 3 contours L7 L14 L18 L42 L43 L44 L45 | L20 L24 L28 L46 L47 L48 L49 bodies 2
fillet "Fillet1" radius 3.5 4 edges at (-2, 16, -1.25) (37, 16, -1.25) (-2, -1, -1.25) (37, -1, -1.25) on bodies 2
fillet "Fillet2" radius 2.5 4 edges at (-2, -4.5, -1.25) (37, -4.5, -1.25) (37, 19.5, -1.25) (-2, 19.5, -1.25) on bodies 2
move_body "Move2" bodies 2 to x (1, 0, 0) y (0, 1, 0) z (0, 0, 1) at (0, -28, 0)
hidden bodies 1
named bodies: "Microphone", "MicrophoneHolder1", "Holder1", "MicrophoneHolder2"
